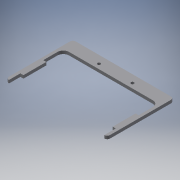
# Autodesk Inventor part: shovel
Saved by Autodesk Inventor 2017.2 (Build 212233000, 233)
## iProperties
Created: 2017-09-14
Part Number: shovel
Material: Generic
Document SubType Name: Modeling
Designer: Nic
Density: 1 g/cm^3
Appearance: Default
Author: Nic
Autodesk Inventor part; units mm, degrees
ref_plane "YZ Plane" through (0, 0, 0) normal (1, 0, 0) x (0, 1, 0)
ref_plane "XZ Plane" through (0, 0, 0) normal (0, 1, 0) x (-1, 0, 0)
ref_plane "XY Plane" through (0, 0, 0) normal (0, 0, 1) x (1, 0, 0)
sketch "Sketch1" plane through (0, 0, 0) normal (0, 0, 1) x (1, 0, 0)
  line L0 (-50, 70) -> (50, 70)
  line L1 (50, 0) -> (-50, 0)
  line L2 (0, 0) -> (0, 70) construction
  circle A0 centre (-17.5, 62) radius 1.6
  circle A1 centre (17.5, 62) radius 1.6
  arc A2 (-50, 70) -> (-53, 67) centre (-50, 67) ccw
  arc A3 (-53, 3) -> (-50, 0) centre (-50, 3) ccw
  arc A4 (53, 67) -> (50, 70) centre (50, 67) ccw
  arc A5 (50, 0) -> (53, 3) centre (50, 3) ccw
  line L3 (53, 67) -> (53, 3)
  line L4 (53, 20) -> (53, 3)
  line L5 (-53, 67) -> (-53, 3)
  line L6 (-53, 20) -> (-53, 3)
  point P0 (53, 45)
  point P1 (-53, 45)
  dimension "d11" = 70
  dimension "d20" = 3
  dimension "d22" = 3.2
  dimension "d23" = 8
  dimension "d24" = 35
  dimension "d31" = 106
  constraints: 14 end point, 10 tangent, 8 point on circle, 6 centre point, 3 equal radius, 3 perpendicular, 2 midpoint, 2 point on line, 2 symmetric about line, 1 collinear, 1 horizontal, 1 parallel, 1 other
  measures "d11" distance between parallel lines of L1 L0
  measures "d20" radius of A2
  measures "d22" diameter of A0
  measures "d23" distance from line of L0 A0.centre
  measures "d24" distance of A1.centre A0.centre
  measures "d31" distance between parallel lines of L4 L6
extrude "Extrusion1" add sketch "Sketch1" along normal blind 3.175
sketch "Sketch2" plane through (0, 0, 3.175) normal (0, 0, 1) x (1, 0, 0)
  line L0 (-44, 57) -> (0, 57)
  line L1 (0, 0) -> (0, 57) construction
  line L2 (44, 57) -> (0, 57)
  line L3 (-50, -5) -> (50, -5)
  line L4 (-50, 0) -> (50, 0) construction
  arc A0 (50, 51) -> (44, 57) centre (44, 51) ccw
  arc A1 (-44, 57) -> (-50, 51) centre (-44, 51) ccw
  line L5 (50, 36) -> (46.8, 36)
  line L6 (46.8, 36) -> (46.8, 12)
  line L7 (46.8, 12) -> (50, 12)
  line L8 (-50, 36) -> (-46.8, 36)
  line L9 (-46.8, 36) -> (-46.8, 12)
  line L10 (-46.8, 12) -> (-50, 12)
  line L11 (50, -5) -> (50, 12)
  line L12 (50, 36) -> (50, 51)
  line L13 (-50, -5) -> (-50, 12)
  line L14 (-50, 36) -> (-50, 51)
  point P0 (47.5, 57)
  point P1 (-47.5, 57)
  dimension "d14" = 57
  dimension "d17" = 62
  dimension "d33" = 6
  dimension "d35" = 36
  dimension "d36" = 12
  dimension "d37" = 100
  dimension "d38" = 3.2
  constraints: 28 end point, 6 symmetric about line, 6 tangent, 4 point on circle, 3 horizontal, 3 perpendicular, 3 vertical, 2 centre point, 2 point on line, 1 equal radius
  measures "d14" distance between parallel lines of L4 L2
  measures "d17" distance between parallel lines of L0 L3
  measures "d33" radius of A0
  measures "d35" distance between parallel lines of L4 L5
  measures "d36" distance between parallel lines of L4 L7
  measures "d37" distance between parallel lines of L14 L12
  measures "d38" distance between parallel lines of L13 L9
extrude "Extrusion2" cut sketch "Sketch2" against normal blind 6
body "Solid1"
